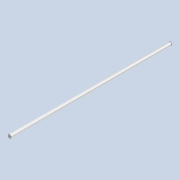
# Autodesk Inventor part: barra
Saved by Autodesk Inventor 2021 (Build 250183000, 183)
## iProperties
Created: 2021-04-15
Part Number: barra
Material: Acero inoxidable AISI 304
Document SubType Name: Modeling
Designer: leo7s
Density: 8 g/cm^3
Appearance: Cromo - Satinado
Mass: 1277.55 g
Surface Area: 427.618 cm^2
Volume: 159.694 cm^3
Author: leo7s
Autodesk Inventor part; units mm, degrees
ref_plane "YZ Plane" through (0, 0, 0) normal (1, 0, 0) x (0, 1, 0)
ref_plane "XZ Plane" through (0, 0, 0) normal (0, 1, 0) x (-1, 0, 0)
ref_plane "XY Plane" through (0, 0, 0) normal (0, 0, 1) x (1, 0, 0)
sketch "Boceto2" plane through (0, 0, 0) normal (0, 0, 1) x (1, 0, 0)
  circle A0 centre (0, 0) radius 7.9375
  dimension "d0" = 15.875
  constraints: 1 centre point, 1 coincident
  measures "d0" diameter of A0
extrude "Extrusión1" add sketch "Boceto2" against normal blind 815
sketch "Boceto3" plane through (0, 0, 0) normal (0, 0, 1) x (1, 0, 0)
  circle A0 centre (0, 0) radius 7.9375 projected
extrude "Extrusión2" add sketch "Boceto3" along normal blind 4
sketch "Boceto6" plane through (0, 0, 4) normal (0, 0, 1) x (1, 0, 0)
  circle A0 centre (0, 0) radius 3
  dimension "d15" = 6
  constraints: 1 centre point, 1 coincident
  measures "d15" diameter of A0
sketch "Boceto7" plane through (0, 0, -815) normal (0, 0, -1) x (-1, 0, 0)
  circle A0 centre (0, 0) radius 3
  dimension "d16" = 6
  constraints: 1 centre point, 1 coincident
  measures "d16" diameter of A0
hole "Agujero1" at (0, 0, -815) direction (0, 0, 1) diameter 6 depth 12 tip angle 118
hole "Agujero2" at (0, 0, 4) direction (0, 0, -1) diameter 6 depth 12 tip angle 118
thread "Rosca3" size "M6x1" class "6H" standard "ANSI Metric M Profile" length 10
thread "Rosca5" size "M6x1" class "6H" standard "ANSI Metric M Profile" length 10
